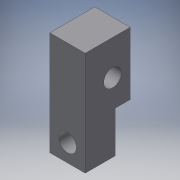
# Autodesk Inventor part: Base_encoder
Saved by Autodesk Inventor 2019 (Build 230136000, 136)
## iProperties
Created: 2018-11-27
Part Number: Base_encoder
Material: Generic
Document SubType Name: Modeling
Designer: Andres
Density: 1 g/cm^3
Appearance: Default
Author: Andres
Autodesk Inventor part; units mm, degrees
ref_plane "YZ Plane" through (0, 0, 0) normal (1, 0, 0) x (0, 1, 0)
ref_plane "XZ Plane" through (0, 0, 0) normal (0, 1, 0) x (-1, 0, 0)
ref_plane "XY Plane" through (0, 0, 0) normal (0, 0, 1) x (1, 0, 0)
sketch "Sketch1" plane through (0, 0, 0) normal (0, 0, 1) x (1, 0, 0)
  circle A0 centre (25, 0) radius 1.5 projected
  line L0 (30, 7.2167) -> (20.6, 7.2167)
  line L1 (30, 10.2167) -> (20.6, 10.2167)
  line L2 (22, -3) -> (28, -3) projected
  line L3 (28, -3) -> (22, -3)
  line L4 (22, -3) -> (22, 14.6155)
  line L5 (22, 14.6155) -> (28, 14.6155)
  line L6 (28, 14.6155) -> (28, -3)
  point P0 (0, 0)
  constraints: 12 end point, 3 horizontal, 2 parallel, 1 perpendicular, 4 other
extrude "Extrusion1" add sketch "Sketch1" along normal blind 5.08 and the other way blind 2.54
sketch "Sketch2" plane through (28, -3, 5.08) normal (1, 0, 0) x (0, 0, -1)
  line L0 (5.08, -1) -> (5.08, 7) projected
  circle A0 centre (4.6338, 11.7167) radius 1.5 projected
  line L1 (5.08, 7) -> (7.62, 7)
  line L2 (7.62, 17.6155) -> (7.62, 0) projected
  line L3 (7.62, 7) -> (7.62, 0)
  line L4 (7.62, 0) -> (5.08, 0)
  line L5 (7.62, 0) -> (0, 0) projected
  line L6 (5.08, 0) -> (5.08, 7)
  point P0 (5.08, 3)
  constraints: 8 end point, 3 point on line, 2 collinear, 1 horizontal, 1 other
extrude "Extrusion2" cut sketch "Sketch2" against normal blind 7.62
body "Solid1"
